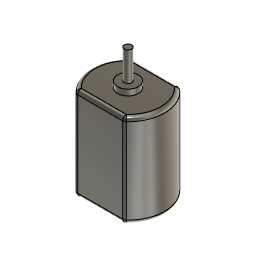
Motorino DC 3V v3 (Autodesk Fusion 360 design; units mm, degrees)
Autodesk Fusion 360 part; units mm, degrees
sketch "Schizzo1" plane through (0, 0, 0) normal (0, 0, 1) x (1, 0, 0)
  circle A0 centre (0, 0) radius 1
  dimension "d1" = 2
  constraint coincident A0.centre origin
  measures "d1" diameter of A0
extrude "Estrudi1" add sketch "Schizzo1" along normal blind 37.9
sketch "Schizzo2" plane through (0, 0, 0) normal (0, 1, 0) x (1, 0, 0)
sketch "Schizzo3" plane through (0, 0, 0) normal (0, 0, 1) x (1, 0, 0)
  line L0 (-2.9326, -3.8) -> (2.9326, -3.8)
  arc A0 (2.9326, -3.8) -> (-2.9326, -3.8) centre (0, 0) ccw
  point P0 (0, 4.8)
  dimension "d4" = 9.6
  dimension "d6" = 3.8
  dimension "d7" = 8.6
  constraint coincident A0.centre origin
  constraint horizontal L0
  constraint midpoint A0 P0
  measures "d4" diameter of A0
  measures "d6" distance of L0 A0.centre
  measures "d7" distance of L0 P0
extrude "Estrudi2" add sketch "Schizzo3" along normal blind 2.4 from surface at 1
sketch "Schizzo4" plane through (0, 0, 3.4) normal (0, 0, 1) x (-1, 0, 0)
  arc A0 (-2.9326, 3.8) -> (2.9326, 3.8) centre (0, 0) ccw
  line L0 (2.9326, 3.8) -> (-2.9326, 3.8)
  circle A1 centre (0, 0) radius 1
  line L1 (6.4622, -7.5) -> (-6.4622, -7.5)
  line L2 (-6.4622, 7.5) -> (6.4622, 7.5)
  arc A2 (-6.4622, 7.5) -> (-6.4622, -7.5) centre (0, 0) ccw
  arc A3 (6.4622, -7.5) -> (6.4622, 7.5) centre (0, 0) ccw
  dimension "d11" = 19.8
  dimension "d12" = 7.5
  dimension "d21" = 15
  constraint horizontal L1
  constraint horizontal L2
  constraint coincident A0.centre A1.centre
  constraint coincident L1.start A2
  constraint concentric A2 A3
  measures "d11" diameter of A2
  measures "d12" distance of A0.centre L1
  measures "d21" distance of L1 L2
extrude "Estrudi3" add sketch "Schizzo4" along normal blind 25 contours A0 L0 | L1 L2 A2 A3
sketch "Schizzo5" plane through (0, 0, 28.4) normal (0, 0, 1) x (-1, 0, 0)
  circle A0 centre (0, 0) radius 1
  arc A1 (-6.4622, 7.5) -> (-6.4622, -7.5) centre (0, 0) ccw
  line L0 (-6.4622, -7.5) -> (6.4622, -7.5)
  arc A2 (6.4622, -7.5) -> (6.4622, 7.5) centre (0, 0) ccw
  line L1 (6.4622, 7.5) -> (-6.4622, 7.5)
  circle A3 centre (0, 0) radius 2.8
  dimension "d16" = 5.6
  constraint concentric A0 A3
  measures "d16" diameter of A3
extrude "Estrudi4" add sketch "Schizzo5" along normal blind 1.6 contours A3
fillet "Raccordo1" radius 1 4 faces at (-2.1541, 7.5, 11.7333) (2.1541, -7.5, 11.7333) (7.7686, 6.1367, 20.0667) (-7.7686, -6.1367, 20.0667)
equation "d9 = 3.4 mm - 1 mm"
equation "d12 = ( 15 / 2 ) * 1 mm"
